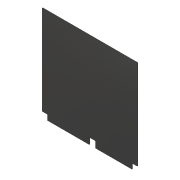
# Autodesk Inventor part: Circuit Board
Saved by Autodesk Inventor 2018.2 (Build 222227000, 227)
## iProperties
Created: 2018-01-23
Part Number: Circuit Board
Material: Glass
Document SubType Name: Modeling
Designer: lopez.xavier
Density: 2.18 g/cm^3
Appearance: Dark Gray
Author: lopez.xavier
Autodesk Inventor part; units mm, degrees
ref_plane "YZ Plane" through (0, 0, 0) normal (1, 0, 0) x (0, 1, 0)
ref_plane "XZ Plane" through (0, 0, 0) normal (0, 1, 0) x (-1, 0, 0)
ref_plane "XY Plane" through (0, 0, 0) normal (0, 0, 1) x (1, 0, 0)
sketch "Sketch1" plane through (0, 0, 0) normal (0, 0, 1) x (1, 0, 0)
  line L0 (0, 0) -> (457.2, 0)
  line L1 (457.2, 0) -> (457.2, 457.2)
  line L2 (457.2, 457.2) -> (0, 457.2)
  line L3 (0, 457.2) -> (0, 0)
  dimension "d0" = 457.2
  dimension "d1" = 457.2
  constraints: 8 end point, 2 parallel, 1 horizontal, 1 perpendicular
  measures "d0" distance of L0.end L1.end
  measures "d1" distance of L1.end L2.end
extrude "Extrusion1" add sketch "Sketch1" along normal blind 2.54
sketch "Sketch2" plane through (0, 0, 2.54) normal (0, 0, 1) x (1, 0, 0)
  line L0 (0, 0) -> (457.2, 0) projected
  line L1 (0, 0) -> (25.4, 0)
  line L2 (25.4, 0) -> (25.4, 25.4)
  line L3 (25.4, 25.4) -> (0, 25.4)
  line L4 (0, 25.4) -> (0, 0)
  line L5 (457.2, 0) -> (431.8, 0)
  line L6 (431.8, 0) -> (431.8, 25.4)
  line L7 (431.8, 25.4) -> (457.2, 25.4)
  line L8 (457.2, 25.4) -> (457.2, 0)
  dimension "d4" = 25.4
  dimension "d5" = 25.4
  dimension "d6" = 25.4
  dimension "d7" = 25.4
  constraints: 16 end point, 4 parallel, 2 horizontal, 2 perpendicular
  measures "d4" distance of L6.end L7.end
  measures "d5" distance of L5.end L6.end
  measures "d6" distance of L1.end L2.end
  measures "d7" distance of L2.end L3.end
extrude "Extrusion2" cut sketch "Sketch2" against normal blind 25.4
sketch "Sketch3" plane through (0, 0, 2.54) normal (0, 0, 1) x (1, 0, 0)
  line L0 (226.06, 0) -> (256.54, 0)
  line L1 (256.54, 0) -> (256.54, 30.48)
  line L2 (256.54, 30.48) -> (226.06, 30.48)
  line L3 (226.06, 30.48) -> (226.06, 0)
  line L4 (25.4, 0) -> (431.8, 0) projected
  line L5 (25.4, 25.4) -> (25.4, 0) projected
  line L6 (431.8, 0) -> (431.8, 25.4) projected
  point P0 (0, 0)
  dimension "d10" = 30.48
  dimension "d11" = 30.48
  dimension "d12" = 0
  dimension "d16" = 175.26
  constraints: 8 end point, 2 parallel, 1 horizontal, 1 perpendicular
  measures "d10" distance of L2.end L1.end
  measures "d11" distance of L0.end L1.end
  measures "d12" distance between parallel lines of L4 L0
  measures "d16" distance between parallel lines of L6 L1
extrude "Extrusion3" cut sketch "Sketch3" against normal blind 25.4
body "Solid1"
